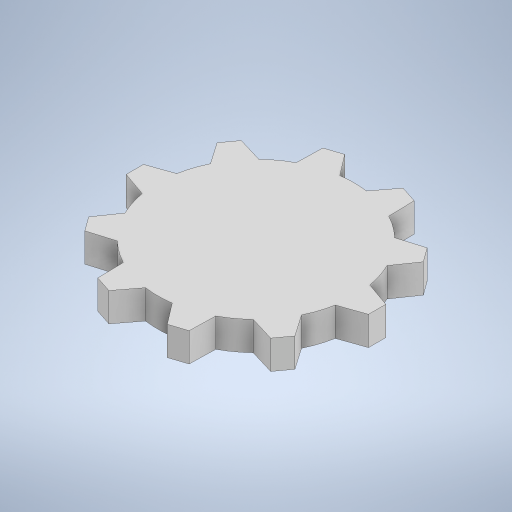
# Autodesk Inventor part: Wrist Sprocket
Saved by Autodesk Inventor 2024 (Build 280153000, 153)
## iProperties
Created: 2023-06-27
Part Number: Wrist Sprocket
Material: Generic
Document SubType Name: Modeling
Designer: t205b
Density: 1 g/cm^3
Appearance: Default
Author: t205b
Autodesk Inventor part; units mm, degrees
ref_plane "YZ Plane" through (0, 0, 0) normal (1, 0, 0) x (0, 1, 0)
ref_plane "XZ Plane" through (0, 0, 0) normal (0, 1, 0) x (-1, 0, 0)
ref_plane "XY Plane" through (0, 0, 0) normal (0, 0, 1) x (1, 0, 0)
sketch "Sketch1" plane through (0, 0, 0) normal (0, 1, 0) x (-1, 0, 0)
  circle A0 centre (0, 0) radius 17
  line L0 (16.7332, -3) -> (21, -1.5)
  line L1 (21, -1.5) -> (21, 1.5)
  line L2 (21, 1.5) -> (16.7332, 3)
  line L3 (15.3008, 7.4085) -> (17.871, 11.13)
  line L4 (17.871, 11.13) -> (16.1077, 13.557)
  line L5 (16.1077, 13.557) -> (11.7741, 12.2626)
  line L6 (8.024, 14.9872) -> (7.9159, 19.5087)
  line L7 (7.9159, 19.5087) -> (5.0628, 20.4357)
  line L8 (5.0628, 20.4357) -> (2.3177, 16.8413)
  line L9 (-2.3177, 16.8413) -> (-5.0628, 20.4357)
  line L10 (-5.0628, 20.4357) -> (-7.9159, 19.5087)
  line L11 (-7.9159, 19.5087) -> (-8.024, 14.9872)
  line L12 (-11.7741, 12.2626) -> (-16.1077, 13.557)
  line L13 (-16.1077, 13.557) -> (-17.871, 11.13)
  line L14 (-17.871, 11.13) -> (-15.3008, 7.4085)
  line L15 (-16.7332, 3) -> (-21, 1.5)
  line L16 (-21, 1.5) -> (-21, -1.5)
  line L17 (-21, -1.5) -> (-16.7332, -3)
  line L18 (-15.3008, -7.4085) -> (-17.871, -11.13)
  line L19 (-17.871, -11.13) -> (-16.1077, -13.557)
  line L20 (-16.1077, -13.557) -> (-11.7741, -12.2626)
  line L21 (-8.024, -14.9872) -> (-7.9159, -19.5087)
  line L22 (-7.9159, -19.5087) -> (-5.0628, -20.4357)
  line L23 (-5.0628, -20.4357) -> (-2.3177, -16.8413)
  line L24 (2.3177, -16.8413) -> (5.0628, -20.4357)
  line L25 (5.0628, -20.4357) -> (7.9159, -19.5087)
  line L26 (7.9159, -19.5087) -> (8.024, -14.9872)
  line L27 (11.7741, -12.2626) -> (16.1077, -13.557)
  line L28 (16.1077, -13.557) -> (17.871, -11.13)
  line L29 (17.871, -11.13) -> (15.3008, -7.4085)
  dimension "d0" = 34
  dimension "d1" = 3
  dimension "d2" = 6
  dimension "d3" = 4
  dimension "d4" = 109.369
  dimension "d5" = 109.369
  dimension "d8" = 360
  constraints: 60 end point, 2 point on circle, 1 centre point, 1 coincident, 1 equal length, 1 vertical, 71 other
  measures "d0" diameter of A0
  measures "d1" distance of L0.end L1.end
  measures "d2" distance of L2.end L0.start
  measures "d3" distance edge to line of A0 L1
  measures "d4" angle of L2 L1
  measures "d5" angle of L0 L1
extrude "Extrusion1" add sketch "Sketch1" along normal blind 5
equation "\"d4\" = d5"
body "Solid1"
